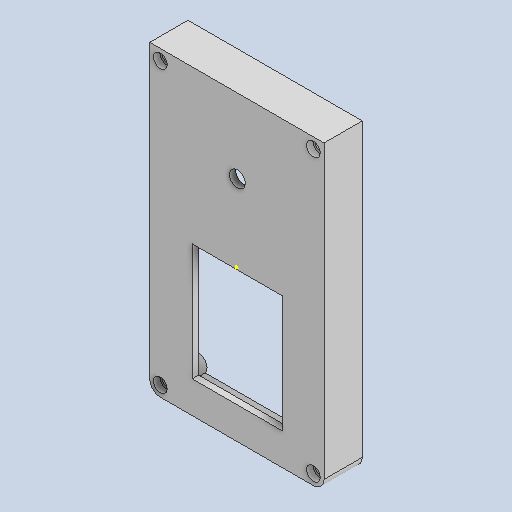
# Autodesk Inventor part: toppcb
Saved by Autodesk Inventor 2026.2 (Build 302298000, 298)
## iProperties
Created: 2026-04-10
Part Number: toppcb
Material: Generic
Document SubType Name: Modeling
Designer: Fork
Density: 1 g/cm^3
Appearance: Default
Author: Fork
Autodesk Inventor part; units mm, degrees
ref_plane "YZ Plane" through (0, 0, 0) normal (1, 0, 0) x (0, 1, 0)
ref_plane "XZ Plane" through (0, 0, 0) normal (0, 1, 0) x (-1, 0, 0)
ref_plane "XY Plane" through (0, 0, 0) normal (0, 0, 1) x (1, 0, 0)
sketch "Sketch1" plane through (0, 0, 0) normal (0, 0, 1) x (1, 0, 0)
  arc A0 (-41, -66.05) -> (-36, -71.05) centre (-36, -66.05) ccw projected
  line L0 (-36, -71.05) -> (36, -71.05) projected
  arc A1 (36, -71.05) -> (41, -66.05) centre (36, -66.05) ccw projected
  line L1 (41, -66.05) -> (41, 86.95) projected
  line L2 (20, 69.05) -> (33.3542, 69.05) projected
  arc A2 (33.3542, 69.05) -> (39, 63.4042) centre (36, 66.05) ccw projected
  line L3 (39, 63.4042) -> (39, -63.4042) projected
  arc A3 (39, -63.4042) -> (33.3542, -69.05) centre (36, -66.05) ccw projected
  line L4 (33.3542, -69.05) -> (-33.3542, -69.05) projected
  arc A4 (-33.3542, -69.05) -> (-39, -63.4042) centre (-36, -66.05) ccw projected
  line L5 (-39, -63.4042) -> (-39, 63.4042) projected
  arc A5 (-39, 63.4042) -> (-33.3542, 69.05) centre (-36, 66.05) ccw projected
  line L6 (-33.3542, 69.05) -> (-20, 69.05) projected
  line L7 (-20, 69.05) -> (-20, 73.05) projected
  circle A6 centre (-36, -66.05) radius 2.1 projected
  line L8 (38.6458, 69.05) -> (39, 69.05) projected
  line L9 (39, 69.05) -> (39, 68.6958) projected
  arc A7 (39, 68.6958) -> (38.6458, 69.05) centre (36, 66.05) ccw projected
  circle A8 centre (36, 66.05) radius 2.1 projected
  line L10 (39, -68.6958) -> (39, -69.05) projected
  line L11 (39, -69.05) -> (38.6458, -69.05) projected
  arc A9 (38.6458, -69.05) -> (39, -68.6958) centre (36, -66.05) ccw projected
  circle A10 centre (36, -66.05) radius 2.1 projected
  arc A11 (-39, -68.6958) -> (-38.6458, -69.05) centre (-36, -66.05) ccw projected
  line L12 (-38.6458, -69.05) -> (-39, -69.05) projected
  line L13 (-39, -69.05) -> (-39, -68.6958) projected
  circle A12 centre (-36, 66.05) radius 2.1 projected
  arc A13 (-38.6458, 69.05) -> (-39, 68.6958) centre (-36, 66.05) ccw projected
  line L14 (-39, 68.6958) -> (-39, 69.05) projected
  line L15 (-39, 69.05) -> (-38.6458, 69.05) projected
  line L16 (20, 71.05) -> (-20, 71.05)
  line L17 (-20, 71.05) -> (-20, 69.05)
  line L18 (-20, 69.05) -> (20, 69.05)
  line L19 (20, 69.05) -> (20, 71.05)
  line L20 (20, 69.05) -> (20, 73.05) projected
  line L21 (-41, -66.05) -> (-41, 86.95) projected
  line L22 (20, 71.05) -> (41, 71.05)
  line L23 (41, 71.05) -> (-41, 71.05)
  line L24 (-39, 79.0505) -> (-39, 73.05) projected
  line L25 (34, 89.95) -> (-34, 89.95) projected
  line L26 (39, 73.05) -> (39, 79.0505) projected
  circle A14 centre (-36.5, 81.5) radius 2.1 projected
  circle A15 centre (36.5, 81.5) radius 2.1 projected
  arc A16 (-39, 79.0505) -> (-39, 83.9495) centre (-36.5, 81.5) ccw projected
  line L27 (-39, 84.95) -> (-39, 83.9495) projected
  line L28 (39, 83.9495) -> (39, 84.95) projected
  arc A17 (39, 83.9495) -> (39, 79.0505) centre (36.5, 81.5) ccw projected
  line L29 (-38.5, 86.95) -> (-38.5, -66.05)
  arc A18 (-38.5, -66.05) -> (-36, -68.55) centre (-36, -66.05) ccw
  line L30 (-36, -68.55) -> (36, -68.55)
  arc A19 (36, -68.55) -> (38.5, -66.05) centre (36, -66.05) ccw
  line L31 (38.5, -66.05) -> (38.5, 86.95)
  arc A20 (38.5, 86.95) -> (36, 89.45) centre (36, 86.95) ccw
  line L32 (36, 89.45) -> (-36, 89.45)
  arc A21 (-36, 89.45) -> (-38.5, 86.95) centre (-36, 86.95) ccw
  line L33 (20, 73.05) -> (39, 73.05) projected
  line L34 (-39, 73.05) -> (-20, 73.05) projected
  arc A22 (-34, 89.95) -> (-39, 84.95) centre (-34, 84.95) ccw projected
  arc A23 (39, 84.95) -> (34, 89.95) centre (34, 84.95) ccw projected
  arc A24 (41, 86.95) -> (36, 91.95) centre (36, 86.95) ccw projected
  line L35 (-36, 91.95) -> (36, 91.95) projected
  arc A25 (-36, 91.95) -> (-41, 86.95) centre (-36, 86.95) ccw projected
  point P0 (0, 0)
  point P1 (-20, 71.05)
  point P2 (38.5, 62.9275)
  point P3 (38.5, -62.9275)
  point P4 (32.8775, -68.55)
  point P5 (-32.8775, -68.55)
  point P6 (-38.5, -62.9275)
  point P7 (-38.5, 62.9275)
  dimension "d32" = 2.5
  constraints: 20 end point, 8 point on circle, 4 centre point, 2 horizontal, 2 parallel, 1 collinear, 1 perpendicular, 1 point on line, 4 other
  measures "d32" distance between parallel lines of L21 L29
extrude "Extrusion1" add sketch "Sketch1" along normal blind 15 contours L21 L23 L29 A5 L5 A4 A18 L30 L4 A3 A19 L31 L3 A2 L22 L1 A1 L0 A0 | L23 L7 L6 A5 L29 | L16 L19 L18 L7 | L29 A4 L5 A5 | L22 L31 A2 L2 L19 | A4 L30 A18 L29 | L30 A3 L4 A4 | A2 L3 A3 L31 | A3 L31 A19 L30
sketch "Sketch2" plane through (0, 0, 15) normal (0, 0, 1) x (1, 0, 0)
  line L0 (39, 63.4042) -> (39, -63.4042) projected
  line L1 (-41, 71.05) -> (-41, -66.05) projected
  arc A0 (-41, -66.05) -> (-36, -71.05) centre (-36, -66.05) ccw projected
  line L2 (-36, -71.05) -> (36, -71.05) projected
  arc A1 (36, -71.05) -> (41, -66.05) centre (36, -66.05) ccw projected
  line L3 (41, -66.05) -> (41, 71.05) projected
  line L4 (41, 71.05) -> (-41, 71.05) projected
  line L5 (-33.3542, 69.05) -> (33.3542, 69.05) projected
  arc A2 (33.3542, 69.05) -> (38.5, 62.9275) centre (36, 66.05) ccw projected
  arc A3 (38.5, -62.9275) -> (32.8775, -68.55) centre (36, -66.05) ccw projected
  arc A4 (-32.8775, -68.55) -> (-38.5, -62.9275) centre (-36, -66.05) ccw projected
  arc A5 (-38.5, 62.9275) -> (-33.3542, 69.05) centre (-36, 66.05) ccw projected
  arc A6 (-38.6458, 69.05) -> (-39, 68.6958) centre (-36, 66.05) ccw projected
  line L6 (-39, 68.6958) -> (-39, 69.05) projected
  line L7 (-39, 69.05) -> (-38.6458, 69.05) projected
  circle A7 centre (-36, 66.05) radius 2.1 projected
  arc A8 (-39, -68.6958) -> (-38.6458, -69.05) centre (-36, -66.05) ccw projected
  line L8 (-38.6458, -69.05) -> (-39, -69.05) projected
  line L9 (-39, -69.05) -> (-39, -68.6958) projected
  circle A9 centre (36, -66.05) radius 2.1 projected
  line L10 (39, -68.6958) -> (39, -69.05) projected
  line L11 (39, -69.05) -> (38.6458, -69.05) projected
  arc A10 (38.6458, -69.05) -> (39, -68.6958) centre (36, -66.05) ccw projected
  circle A11 centre (36, 66.05) radius 2.1 projected
  line L12 (38.6458, 69.05) -> (39, 69.05) projected
  line L13 (39, 69.05) -> (39, 68.6958) projected
  arc A12 (39, 68.6958) -> (38.6458, 69.05) centre (36, 66.05) ccw projected
  circle A13 centre (-36, -66.05) radius 2.1 projected
  line L14 (38.5, 62.9275) -> (38.5, -62.9275) projected
  line L15 (32.8775, -68.55) -> (-32.8775, -68.55) projected
  line L16 (-38.5, -62.9275) -> (-38.5, 62.9275) projected
  point P0 (0, 0)
extrude "Extrusion2" add sketch "Sketch2" along normal blind 3 contours L4 L3 A1 L2 A0 L1 | L5 A2 L14 A3 L15 A4 L16 A5 | A6 L6 L7 | A7 | A8 L8 L9 | A9 | L10 L11 A10 | A11 | L12 L13 A12 | A13
sketch "Sketch3" plane through (0, 0, 18) normal (0, 0, 1) x (1, 0, 0)
  line L0 (21.5, -1.05) -> (-21, -1.05)
  line L1 (-21, -1.05) -> (-21, -56.05)
  line L2 (-21, -56.05) -> (21.5, -56.05)
  line L3 (21.5, -56.05) -> (21.5, -1.05)
  line L4 (21.5, -1.05) -> (-21, -56.05) construction
  line L5 (-21, -1.05) -> (21.5, -56.05) construction
  line L6 (-36, -71.05) -> (36, -71.05) projected
  line L7 (41, -66.05) -> (41, 71.05) projected
  line L8 (41, 71.05) -> (-41, 71.05) projected
  line L9 (-41, 71.05) -> (-41, -66.05) projected
  line L10 (41, -66.05) -> (-41, -66.05)
  line L11 (-41, -66.05) -> (-41, 0)
  line L12 (-41, 0) -> (41, 0)
  line L13 (41, 0) -> (41, -66.05)
  line L14 (0.25, -66.05) -> (0.25, 0)
  circle A0 centre (0.25, 36.05) radius 3.75
  point P0 (0, 0)
  point P1 (0.25, -28.55)
  point P2 (-21, -28.55)
  point P3 (41, -33.025)
  dimension "d4" = 42.5
  dimension "d5" = 55
  dimension "d6" = 15
  dimension "d9" = 40.75
  dimension "d10" = 71.05
  dimension "d11" = 19.5
  dimension "d14" = 7.5
  dimension "d15" = 35
  dimension "d16" = 40.75
  constraints: 22 end point, 4 midpoint, 4 parallel, 3 perpendicular, 3 point on line, 2 horizontal, 1 centre point
  measures "d4" distance of L2.end L1.end
  measures "d5" distance of L1.end L0.end
  measures "d6" distance between parallel lines of L6 L2
  measures "d9" distance between parallel lines of L13 L14
  measures "d10" distance between parallel lines of L8 L12
  measures "d11" distance from line of point (41, -33.025) L3
  measures "d14" diameter of A0
  measures "d15" distance from line of L8 A0.centre
  measures "d16" distance from line of L7 A0.centre
extrude "Extrusion3" cut sketch "Sketch3" against normal blind 3 contours L3 L2 L14 L0 | L14 L2 L1 L0 | A0
sketch "Sketch6" plane through (0, 0, 18) normal (0, 0, 1) x (1, 0, 0)
  point P0 (0, 0)
sketch "Sketch7" plane through (0, 0, 18) normal (0, 0, 1) x (1, 0, 0)
  circle A0 centre (-36, -66.05) radius 2.1 projected
  circle A1 centre (36, -66.05) radius 2.1 projected
  circle A2 centre (36, 66.05) radius 2.1 projected
  circle A3 centre (-36, 66.05) radius 2.1 projected
  circle A4 centre (-36, -66.05) radius 3.25
  circle A5 centre (36, -66.05) radius 3.25
  circle A6 centre (-36, 66.05) radius 3.25
  circle A7 centre (36, 66.05) radius 2.1 projected
  circle A8 centre (36, 66.05) radius 3.25
  point P0 (0, 0)
  dimension "d26" = 6.5
  dimension "d27" = 6.5
  dimension "d28" = 6.5
  dimension "d29" = 6.5
  constraints: 4 centre point, 4 coincident
  measures "d26" diameter of A4
  measures "d27" diameter of A5
  measures "d28" diameter of A6
  measures "d29" diameter of A8
extrude "Extrusion6" cut sketch "Sketch7" against normal blind 3 contours A0 | A1 | A2 | A3 | A4 | A5 | A6 | A8
body "Solid1"
